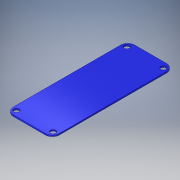
# Autodesk Inventor part: PCB
Saved by Autodesk Inventor 2019 (Build 230136000, 136)
## iProperties
Created: 2020-02-13
Part Number: PCB
Material: Generic
Document SubType Name: Modeling
Designer: close
Density: 1 g/cm^3
Appearance: Blue - Wall Paint - Glossy
Author: close
Autodesk Inventor part; units mm, degrees
ref_plane "YZ Plane" through (0, 0, 0) normal (1, 0, 0) x (0, 1, 0)
ref_plane "XZ Plane" through (0, 0, 0) normal (0, 1, 0) x (-1, 0, 0)
ref_plane "XY Plane" through (0, 0, 0) normal (0, 0, 1) x (1, 0, 0)
sketch "Sketch1" plane through (0, 0, 0) normal (0, 1, 0) x (-1, 0, 0)
  line L0 (0, 0) -> (39.5, 0)
  line L1 (39.5, 0) -> (39.5, -104.35)
  line L2 (39.5, -104.35) -> (0, -104.35)
  line L3 (0, -104.35) -> (0, 0)
  dimension "d0" = 104.35
  dimension "d1" = 39.5
  constraints: 8 end point, 2 parallel, 1 horizontal, 1 perpendicular
  measures "d0" distance of L0.end L1.end
  measures "d1" distance of L1.end L2.end
extrude "Extrusion1" add sketch "Sketch1" along normal blind 1.2
fillet "Fillet1" radius 6 4 edges at (0, 0.6, 0) (-39.5, 0.6, 0) (0, 0.6, -104.35) (-39.5, 0.6, -104.35)
sketch "Sketch2" plane through (0, 0, 0) normal (0, -1, 0) x (1, 0, 0)
  line L0 (-35.5, -99.675) -> (-4, -99.675) construction
  line L1 (-4, -99.675) -> (-4, -4.675) construction
  line L2 (-4, -4.675) -> (-35.5, -4.675) construction
  line L3 (-35.5, -4.675) -> (-35.5, -99.675) construction
  line L4 (0, -98.35) -> (0, -6) construction
  line L5 (-39.5, -6) -> (-39.5, -98.35) construction
  line L6 (-6, 0) -> (-33.5, 0) construction
  line L7 (-33.5, -104.35) -> (-6, -104.35) construction
  point P0 (0, 0)
  dimension "d5" = 95
  dimension "d6" = 31.5
  dimension "d7" = 39.5
  dimension "d8" = 4
  dimension "d9" = 104.35
  dimension "d10" = 4.675
  constraints: 8 end point, 4 coincident, 2 parallel, 1 horizontal, 1 perpendicular
  measures "d5" distance between parallel lines of L2 L0
  measures "d6" distance between parallel lines of L1 L3
  measures "d7" distance between parallel lines of L4 L5
  measures "d8" distance between parallel lines of L5 L3
  measures "d9" distance between parallel lines of L6 L7
  measures "d10" distance between parallel lines of L7 L0
hole "Hole1" at (-35.5, 0, -99.675) at (-4, 0, -99.675) at (-4, 0, -4.675) at (-35.5, 0, -4.675) direction (0, 1, 0) diameter 4.5 depth 1.2 clearance for "Flat Head Machine Screw" size "M4" standard "Ansi Metric M Profile"
equation "\"d8\" = -0.5 * d6 + 0.5 * d7"
equation "\"d10\" = -0.5 * d5 + 0.5 * d9"
body "Solid1"
